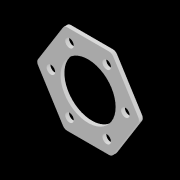
# Autodesk Inventor part: TorsoSpacer
Saved by Autodesk Inventor 2020 (Build 240168000, 168)
## iProperties
Created: 2020-06-07
Part Number: TorsoSpacer
Material: Generic
Document SubType Name: Sheet Metal
Designer: valer
Density: 1 g/cm^3
Sheet Metal Rule: Default
Appearance: Default
Author: valer
Autodesk Inventor part; units mm, degrees
ref_plane "YZ Plane" through (0, 0, 0) normal (1, 0, 0) x (0, 1, 0)
ref_plane "XZ Plane" through (0, 0, 0) normal (0, 1, 0) x (-1, 0, 0)
ref_plane "XY Plane" through (0, 0, 0) normal (0, 0, 1) x (1, 0, 0)
sketch "Base" plane through (0, 0, 0) normal (0, 0, 1) x (1, 0, 0)
  circle A0 centre (0, -88.9) radius 37
  circle A1 centre (-25, -45.5987) radius 5.75
  circle A2 centre (-50, -88.9) radius 5.75
  circle A3 centre (-25, -132.2013) radius 5.75
  circle A4 centre (25, -132.2013) radius 5.75
  circle A5 centre (50, -88.9) radius 5.75
  circle A6 centre (25, -45.5987) radius 5.75
  line L0 (31.8195, -149.0871) -> (69.4286, -88.9)
  line L1 (-31.8195, -149.0871) -> (31.8195, -149.0871)
  line L2 (-69.4286, -88.9) -> (-31.8195, -149.0871)
  circle A7 centre (0, -88.9) radius 50 construction
  line L3 (-50, -88.9) -> (50, -88.9) construction
  line L4 (31.8195, -28.7129) -> (69.4286, -88.9)
  line L5 (-31.8195, -28.7129) -> (31.8195, -28.7129)
  line L6 (-69.4286, -88.9) -> (-31.8195, -28.7129)
  point P0 (0, 0)
  point P1 (0, 0)
  point P2 (33.6847, -146.102)
  point P3 (61.1047, -102.2209)
  point P4 (-28.2996, -149.0871)
  point P5 (28.2996, -149.0871)
  point P6 (-61.1047, -102.2209)
  point P7 (-33.6847, -146.102)
  point P8 (33.6847, -31.698)
  point P9 (61.1047, -75.5791)
  point P10 (-28.2996, -28.7129)
  point P11 (28.2996, -28.7129)
  point P12 (-61.1047, -75.5791)
  point P13 (-33.6847, -31.698)
  dimension "d0" = 74
  dimension "d1" = 11.5
  dimension "d2" = 13
  dimension "d3" = 60.1871
  dimension "d4" = 122
  dimension "d5" = 122
  dimension "d6" = 60.1871
  dimension "d7" = 11.7689
  dimension "d8" = 105.9886
  dimension "d9" = 11.7689
  dimension "d10" = 14.118
  dimension "d11" = 16.4764
  dimension "d12" = 60.6249
  dimension "d13" = 2.985
  dimension "d14" = 14.7314
  dimension "d15" = 60.6237
  dimension "d16" = 11.7689
  dimension "d17" = 105.9886
  dimension "d18" = 57.1338
  dimension "d19" = 103.0261
  dimension "d20" = 50.9839
  dimension "d21" = 57.1326
  dimension "d22" = 103.6395
  measures "d0" diameter of A0
  measures "d1" diameter of A6
  measures "d2" radial gap between concentric circles of A7 A0
  measures "d3" distance from line of L1 A0.centre
  measures "d4" angle of L0 L1
  measures "d5" angle of L2 L1
  measures "d6" distance between parallel lines of L5 L3
  measures "d7" distance from line of point (0, 0) L4
  measures "d8" distance from line of point (0, 0) L0
  measures "d9" distance from line of point (0, 0) L6
  measures "d10" distance from line of point (61.105, -75.579) L0
  measures "d11" distance from line of L3.end L4
  measures "d12" distance from line of point (33.685, -31.698) L0
  measures "d13" distance from line of point (28.3, -28.713) L4
  measures "d14" distance from line of A6.centre L4
  measures "d15" distance from line of A4.centre L4
  measures "d16" distance from line of point (0, 0) L4
  measures "d17" distance from line of point (0, 0) L0
  measures "d18" distance from line of A1.centre L4
  measures "d19" distance from line of A3.centre L4
  measures "d20" distance from line of point (-28.3, -28.713) L4
  measures "d21" distance from line of point (-33.685, -31.698) L4
  measures "d22" distance from line of point (-61.105, -75.579) L4
extrude "Plate1" add sketch "Base" along normal blind 5.08
fillet "BaseFilletsFeature" radius 6.35 6 edges at (31.8195, -149.0871, 2.54) (-31.8195, -149.0871, 2.54) (69.4286, -88.9, 2.54) (-69.4286, -88.9, 2.54) (31.8195, -28.7129, 2.54) (-31.8195, -28.7129, 2.54)
equation "\"d5\" = d4"
equation "\"d23\" = Thickness"
equation "\"BendRadius\" = Thickness"
equation "\"BendReliefWidth\" = Thickness"
equation "\"BendReliefDepth\" = 0.5 * Thickness"
equation "\"CornerReliefSize\" = 4 * Thickness"
equation "\"MinimumRemnant\" = 2 * Thickness"
equation "\"TransitionRadius\" = BendRadius"
equation "\"JacobiRadiusSize\" = BendRadius"
equation "\"GapSize\" = Thickness"
equation "\"Thickness\" = 5.08"
body "Solid1"
